ESP32CAM Front (Autodesk Fusion 360 design; units mm, degrees)
Autodesk Fusion 360 part; units mm, degrees
sketch "Sketch2" plane through (0, 0, 0) normal (0, 0, 1) x (1, 0, 0)
  line L0 (14.75, -0.5) -> (-14.75, -0.5)
  line L1 (-14.75, -0.5) -> (-14.75, 0.5)
  line L2 (-14.75, 0.5) -> (14.75, 0.5)
  line L3 (14.75, 0.5) -> (14.75, -0.5)
  line L4 (14.75, -0.5) -> (-14.75, 0.5) construction
  line L5 (-14.75, -0.5) -> (14.75, 0.5) construction
  line L6 (-14.75, 0.5) -> (-13.75, 0.5)
  line L7 (-13.75, 0.5) -> (-13.75, 5.5)
  line L8 (-13.75, 5.5) -> (-14.75, 5.5)
  line L9 (-14.75, 5.5) -> (-14.75, 0.5)
  line L10 (-13.75, 5.5) -> (-13.25, 5.5)
  line L11 (-13.25, 5.5) -> (-13.25, 4.5)
  line L12 (-13.25, 4.5) -> (-13.75, 4.5)
  line L13 (-13.75, 4.5) -> (-13.75, 5.5)
  line L14 (0, 0) -> (0, 15) construction
  line L15 (13.25, 5.5) -> (13.25, 4.5)
  line L16 (14.75, 0.5) -> (13.75, 0.5)
  line L17 (13.75, 5.5) -> (14.75, 5.5)
  line L18 (13.75, 5.5) -> (13.25, 5.5)
  line L19 (14.75, 5.5) -> (14.75, 0.5)
  line L20 (13.75, 4.5) -> (13.75, 5.5)
  line L21 (13.75, 0.5) -> (13.75, 5.5)
  line L22 (13.25, 4.5) -> (13.75, 4.5)
  dimension "d7" = 1
  dimension "d8" = 1
  dimension "d10" = 1
  dimension "d11" = 0.5
  dimension "d12" = 4
  dimension "d13" = 13.75
  constraint perpendicular L0 L1
  constraint parallel L0 L2
  constraint parallel L1 L3
  constraint horizontal L0
  constraint coincident L4 L14.start
  constraint coincident L5 L14.start
  constraint coincident L14.start origin
  constraint horizontal L6
  constraint vertical L7
  constraint horizontal L8
  constraint vertical L9
  constraint horizontal L10
  constraint vertical L11
  constraint horizontal L12
  constraint vertical L13
  constraint perpendicular L2 L14
  constraint symmetric L1.end L14 L2.end
  constraint symmetric L6.end L14 L16.end
  constraint symmetric L7.end L14 L17.start
  constraint symmetric L8.end L14 L17.end
  constraint symmetric L10.end L14 L15.start
  constraint symmetric L11.end L14 L15.end
  constraint symmetric L12.end L14 L20.start
  measures "d7" distance of L0.end L1.end
  measures "d8" distance of L1.end L6.end
  measures "d10" distance of L7.end L12.end
  measures "d11" distance of L7.end L10.end
  measures "d12" distance of L2 L11.end
  measures "d13" horizontal distance of L14.start L6.end
extrude "Extrude1" add sketch "Sketch2" along normal blind 10
equation "d13 = ( 27.5 / 2 ) * 1 mm"
